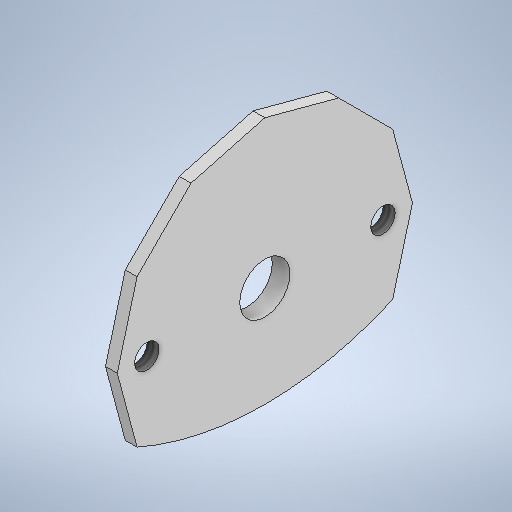
# Autodesk Inventor part: bielle côté 0
Saved by Autodesk Inventor 2025.2 (Build 292293000, 293)
## iProperties
Created: 2026-03-16
Part Number: bielle côté 0
Material: Générique
Document SubType Name: Modeling
Designer: genon
Density: 1 g/cm^3
Appearance: Par défaut
Author: genon
Autodesk Inventor part; units mm, degrees
ref_plane "YZ Plane" through (0, 0, 0) normal (1, 0, 0) x (0, 1, 0)
ref_plane "XZ Plane" through (0, 0, 0) normal (0, 1, 0) x (-1, 0, 0)
ref_plane "XY Plane" through (0, 0, 0) normal (0, 0, 1) x (1, 0, 0)
sketch "Esquisse1" plane through (0, 0, 0) normal (1, 0, 0) x (0, 1, 0)
  circle A0 centre (0, 0) radius 10.95
  circle A1 centre (0, 0) radius 25
  line L0 (0, 25) -> (25, 25)
  line L1 (25, 25) -> (25, 0)
  line L2 (21.6506, 12.5) -> (25, 0)
  line L3 (21.6506, 12.5) -> (12.5, 21.6506)
  line L4 (12.5, 21.6506) -> (0, 25)
  line L5 (0, 0) -> (7.9736, 0)
  line L6 (0, 0) -> (0, 6.25)
  line L7 (21.6506, -12.5) -> (25, 0)
  line L8 (21.6506, -12.5) -> (12.5, -21.6506)
  line L9 (12.5, -21.6506) -> (0, -25)
  line L10 (-21.6506, 12.5) -> (-25, 0)
  line L11 (-21.6506, 12.5) -> (-12.5, 21.6506)
  line L12 (-12.5, 21.6506) -> (0, 25)
  line L13 (-21.6506, -12.5) -> (-25, 0)
  line L14 (-21.6506, -12.5) -> (-12.5, -21.6506)
  line L15 (-12.5, -21.6506) -> (0, -25)
  line L16 (-12.5, 21.6506) -> (-12.5, -21.6506)
  arc A2 (-12.5, 21.6506) -> (-12.5, -21.6506) centre (36.4383, 0) ccw
  dimension "d0" = 21.9
  dimension "d1" = 50
  constraints: 34 end point, 8 symmetric about line, 6 point on circle, 3 centre point, 2 coincident, 2 horizontal, 2 tangent, 2 vertical
  measures "d0" diameter of A0
  measures "d1" diameter of A1
extrude "Extrusion1" add sketch "Esquisse1" along normal blind 2 contours L7 L8 L9 L15 L16 L12 L4 L3 L2 | L16 A2
sketch "Esquisse7" plane through (2, 0, 0) normal (1, 0, 0) x (0, 0, -1)
  circle A0 centre (0, 0) radius 10.95
  circle A1 centre (0, 0) radius 4.25
  constraints: 2 centre point, 2 coincident
extrude "Extrusion6" add sketch "Esquisse7" against normal blind 3
sketch "Esquisse8" plane through (0, 0, 0) normal (-1, 0, 0) x (0, 0, 1)
  line L0 (0, 0) -> (-20, 0)
  line L1 (0, 0) -> (0, 2.8662)
  point P0 (20, 0)
  dimension "d30" = 20
  constraints: 4 end point, 1 coincident, 1 horizontal, 1 symmetric about line, 1 vertical
  measures "d30" distance of L0.start L0.end
hole "Perçage2" at (0, 0, -20) at (0, 0, 20) direction (1, 0, 0) diameter 4.134 end through all thread size "M5x0.8" class "6H" standard "ISO Metric profile"
